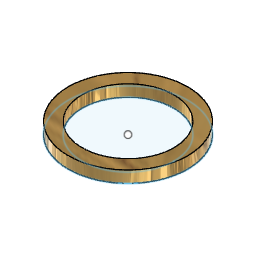
Centering ring v4 (Autodesk Fusion 360 design; units mm, degrees)
Autodesk Fusion 360 part; units mm, degrees
sketch "Sketch1" plane through (0, 0, 0) normal (0, 0, 1) x (1, 0, 0)
  circle A0 centre (17.385, 5) radius 15.75
  circle A1 centre (17.385, 5) radius 20.5
  dimension "d3" = 31.5
  dimension "d4" = 41
  measures "d3" diameter of A0
  measures "d4" diameter of A1
extrude "Extrude1" add sketch "Sketch1" along normal blind 4
